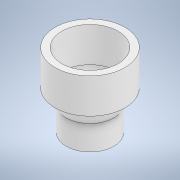
# Autodesk Inventor part: PVC_connector
Saved by Autodesk Inventor 2020.1 (Build 241239000, 239)
## iProperties
Created: 2019-11-10
Part Number: PVC_connector
Material: PVC-Piping
Document SubType Name: Modeling
Designer: Paul Lefeuvre
Density: 1.4 g/cm^3
Appearance: Smooth - White
Author: Paul Lefeuvre
Autodesk Inventor part; units mm, degrees
ref_plane "YZ Plane" through (0, 0, 0) normal (1, 0, 0) x (0, 1, 0)
ref_plane "XZ Plane" through (0, 0, 0) normal (0, 1, 0) x (-1, 0, 0)
ref_plane "XY Plane" through (0, 0, 0) normal (0, 0, 1) x (1, 0, 0)
sketch "Sketch1" plane through (0, 0, 0) normal (0, 0, 1) x (1, 0, 0)
  line L0 (0, 0) -> (35.5, 0)
  line L1 (35.5, 0) -> (35.5, 44)
  line L2 (35.5, 44) -> (0, 44)
  line L3 (0, 44) -> (0, 0)
  line L4 (0, 0) -> (0, -18)
  line L5 (0, -18) -> (25, -18)
  line L6 (25, -18) -> (25, -49)
  line L7 (25, -49) -> (0, -49)
  line L8 (0, -49) -> (0, -18)
  line L9 (35.5, 0) -> (25, -18)
  line L10 (0, 0) -> (44, 0)
  line L11 (44, 0) -> (44, 44)
  line L12 (44, 44) -> (0, 44)
  line L13 (0, 44) -> (0, 0)
  line L14 (0, -18) -> (30, -18)
  line L15 (30, -18) -> (30, -49)
  line L16 (30, -49) -> (0, -49)
  line L17 (0, -49) -> (0, -18)
  line L18 (30, -18) -> (44, 0)
  dimension "d13" = 35.5
  dimension "d14" = 44
  dimension "d15" = 18
  dimension "d16" = 25
  dimension "d17" = 31
  dimension "d18" = 44
  dimension "d19" = 30
  constraints: 38 end point, 8 parallel, 4 horizontal, 4 perpendicular, 1 vertical
  measures "d13" distance of L2.end L1.end
  measures "d14" distance of L1.end L0.end
  measures "d15" distance of L0.start L4.end
  measures "d16" distance of L6.end L7.end
  measures "d17" distance of L5.end L6.end
  measures "d18" distance of L12.end L11.end
  measures "d19" distance of L15.end L16.end
revolve "Revolution1" add sketch "Sketch1" angle 360 about axis through (0, -49, 0) along (0, 1, 0) contours L10 L18 L14 L9 | L1 L12 L11 L10 | L14 L15 L16 L6
body "Solid2"
